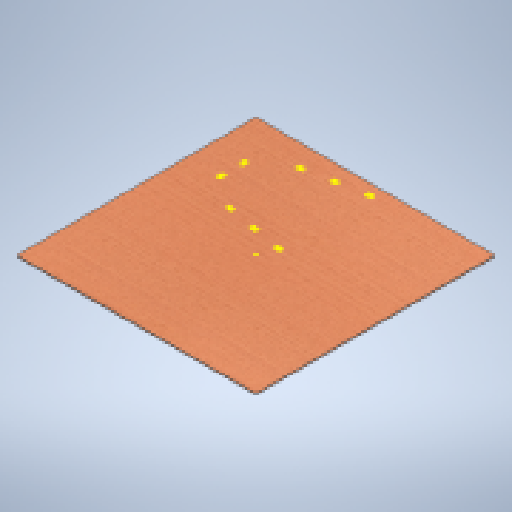
# Autodesk Inventor part: plate
Saved by Autodesk Inventor 2025.2 (Build 292293000, 293)
## iProperties
Created: 2025-04-09
Part Number: plate
Material: Generic
Document SubType Name: Modeling
Designer: abdal
Density: 1 g/cm^3
Appearance: Default
Author: abdal
Autodesk Inventor part; units mm, degrees
ref_plane "YZ Plane" through (0, 0, 0) normal (1, 0, 0) x (0, 1, 0)
ref_plane "XZ Plane" through (0, 0, 0) normal (0, 1, 0) x (-1, 0, 0)
ref_plane "XY Plane" through (0, 0, 0) normal (0, 0, 1) x (1, 0, 0)
sketch "Sketch1" plane through (0, 0, 0) normal (0, 1, 0) x (-1, 0, 0)
  line L0 (198, 200) -> (-198, 200)
  line L1 (-200, 198) -> (-200, -198)
  line L2 (-198, -200) -> (200, -200)
  line L3 (200, -200) -> (200, 198)
  line L4 (200, 200) -> (-200, -200) construction
  line L5 (-200, 200) -> (200, -200) construction
  arc A0 (200, 198) -> (198, 200) centre (198, 198) ccw
  arc A1 (-198, 200) -> (-200, 198) centre (-198, 198) ccw
  arc A2 (-200, -198) -> (-198, -200) centre (-198, -198) ccw
  point P0 (0, 0)
  dimension "d0" = 400
  dimension "d1" = 400
  dimension "d2" = 2
  constraints: 12 end point, 6 point on circle, 6 point on line, 6 tangent, 3 centre point, 2 equal radius, 2 midpoint, 2 parallel, 1 horizontal, 1 perpendicular
  measures "d0" distance of L2.end L4.start
  measures "d1" distance of L4.end L2.end
  measures "d2" radius of A0
extrude "Extrusion1" add sketch "Sketch1" along normal blind 2
sketch "Sketch2" plane through (0, 2, 0) normal (0, 1, 0) x (1, 0, 0)
  circle A0 centre (-89.3419, 163.5375) radius 1.5 projected
  line L0 (-84.9588, 167.383) -> (-94.7977, 165.5953) projected
  line L1 (-94.7977, 165.5953) -> (-93.7251, 159.692) projected
  line L2 (-93.7251, 159.692) -> (-83.8862, 161.4797) projected
  line L3 (-84.9588, 167.383) -> (-83.8862, 161.4797) projected
  circle A1 centre (-144.1798, 123.3441) radius 1.5 projected
  line L4 (-147.1798, 118.3441) -> (-147.1798, 128.3441) projected
  line L5 (-141.1798, 118.3441) -> (-147.1798, 118.3441) projected
  line L6 (-141.1798, 128.3441) -> (-141.1798, 118.3441) projected
  line L7 (-141.1798, 128.3441) -> (-147.1798, 128.3441) projected
  circle A2 centre (-144.1798, 85.8947) radius 1.5 projected
  line L8 (-147.1798, 80.8947) -> (-147.1798, 90.8947) projected
  line L9 (-147.1798, 80.8947) -> (-141.1798, 80.8947) projected
  line L10 (-141.1798, 90.8947) -> (-141.1798, 80.8947) projected
  line L11 (-147.1798, 90.8947) -> (-141.1798, 90.8947) projected
  circle A3 centre (-89.3419, 46.4625) radius 1.5 projected
  circle A4 centre (-89.3419, 46.4625) radius 1.5 projected
  line L12 (-84.9588, 42.617) -> (-94.7977, 44.4047) projected
  line L13 (-84.9588, 42.617) -> (-83.8862, 48.5203) projected
  line L14 (-93.7251, 50.308) -> (-83.8862, 48.5203) projected
  line L15 (-94.7977, 44.4047) -> (-93.7251, 50.308) projected
  circle A5 centre (-40.1474, 37.5241) radius 1.5 projected
  line L16 (-35.7642, 33.6786) -> (-45.6031, 35.4663) projected
  line L17 (-35.7642, 33.6786) -> (-34.6916, 39.5819) projected
  line L18 (-44.5305, 41.3696) -> (-34.6916, 39.5819) projected
  line L19 (-45.6031, 35.4663) -> (-44.5305, 41.3696) projected
  circle A6 centre (9.0472, 28.5857) radius 1.5 projected
  line L20 (13.4304, 24.7402) -> (3.5914, 26.5278) projected
  line L21 (13.4304, 24.7402) -> (14.503, 30.6435) projected
  line L22 (4.6641, 32.4312) -> (14.503, 30.6435) projected
  line L23 (3.5914, 26.5278) -> (4.6641, 32.4312) projected
  circle A7 centre (-40.1474, 172.4759) radius 1.5 projected
  line L24 (-35.7642, 176.3214) -> (-45.6031, 174.5337) projected
  line L25 (-45.6031, 174.5337) -> (-44.5305, 168.6304) projected
  line L26 (-44.5305, 168.6304) -> (-34.6916, 170.4181) projected
  line L27 (-35.7642, 176.3214) -> (-34.6916, 170.4181) projected
  circle A8 centre (9.0472, 181.4143) radius 1.5 projected
  line L28 (13.4304, 185.2598) -> (3.5914, 183.4722) projected
  line L29 (3.5914, 183.4722) -> (4.6641, 177.5688) projected
  line L30 (4.6641, 177.5688) -> (14.503, 179.3565) projected
  line L31 (13.4304, 185.2598) -> (14.503, 179.3565) projected
  point P0 (0, 0)
extrude "Extrusion2" cut sketch "Sketch2" against normal through all contours A0 | A1 | A2 | A3 | A5 | A6 | A7 | A8
body "Solid1"
